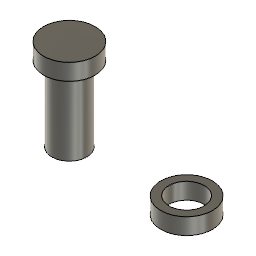
Wheel Connectors (Autodesk Fusion 360 design; units mm, degrees)
Autodesk Fusion 360 part; units mm, degrees
sketch "Sketch1" plane through (0, 0, 0) normal (0, 0, 1) x (1, 0, 0)
  line L0 (0, 0) -> (0, -2.6) construction
  line L1 (0, -2.6) -> (0, -2.2) construction
  line L2 (-1.2894, -2.2) -> (1.2894, -2.2)
  arc A0 (1.2894, -2.2) -> (-1.2894, -2.2) centre (0, 0) ccw
  circle A1 centre (0, 0) radius 7.5
  dimension "d34" = 5.1
  dimension "d36" = 0.4
  dimension "d37" = 15
  constraint coincident L0.start A0.centre
  constraint vertical L0
  constraint parallel L0 L1
  constraint midpoint L1.end L2
  constraint perpendicular L0 L2
  constraint concentric A0 A1
  measures "d34" diameter of A0
  measures "d36" distance of L0.end L1.end
  measures "d37" diameter of A1
extrude "Extrude9" add sketch "Sketch1" along normal blind 32 makes body 1
ref_plane "WorkPlane3" through (0, 0, 32) normal (0, 0, 1) x (1, 0, 0)
sketch "Sketch4" plane through (0, 0, 32) normal (0, 0, 1) x (1, 0, 0)
  circle A0 centre (0, 0) radius 11
  dimension "d41" = 22
  constraint coincident A0.centre origin
  measures "d41" diameter of A0
extrude "Extrude10" add sketch "Sketch4" along normal blind 7 bodies 1
sketch "Sketch5" plane through (0, 0, 0) normal (0, 0, 1) x (1, 0, 0)
  line L0 (0, 0) -> (50, 0) construction
  circle A0 centre (50, 0) radius 7.5
  circle A1 centre (50, 0) radius 11
  dimension "d44" = 50
  dimension "d45" = 15
  dimension "d46" = 22
  constraint coincident L0.start origin
  constraint horizontal L0
  constraint coincident L0.end A0.centre
  constraint concentric A0 A1
  measures "d44" distance of L0.start L0.end
  measures "d45" diameter of A0
  measures "d46" diameter of A1
extrude "Extrude11" add sketch "Sketch5" along normal blind 7 separate body makes body 2
equation "holder_diameter = 15 mm"
equation "hole_diameter = 5.1 mm"
equation "indent_size = 0.4 mm"
equation "washer_height = 10 mm"
equation "metal_pole_height = 15 mm"
equation "wheel_thickness = 24 mm"
equation "wheel_hold_diameter = 8.1 mm"
equation "outside_wheel_cap_diameter = 22 mm"
equation "cap_thickness = 7 mm"
equation "d34 = hole_diameter"
equation "d36 = indent_size"
equation "d37 = holder_diameter"
equation "d38 = metal_pole_height + wheel_thickness - cap_thickness"
equation "d40 = metal_pole_height + wheel_thickness - cap_thickness"
equation "d41 = outside_wheel_cap_diameter"
equation "d42 = cap_thickness"
equation "d45 = holder_diameter"
equation "d46 = outside_wheel_cap_diameter"
equation "d47 = cap_thickness"
